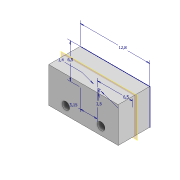
# Autodesk Inventor part: LimitSwitch
Saved by Autodesk Inventor 2022 (Build 260153000, 153)
## iProperties
Created: 2022-11-25
Part Number: LimitSwitch
Material: Generisch
Document SubType Name: Modeling
Designer: alexw
Density: 1 g/cm^3
Appearance: Vorgabe
Author: alexw
Autodesk Inventor part; units mm, degrees
ref_plane "YZ Plane" through (0, 0, 0) normal (1, 0, 0) x (0, 1, 0)
ref_plane "XZ Plane" through (0, 0, 0) normal (0, 1, 0) x (-1, 0, 0)
ref_plane "XY Plane" through (0, 0, 0) normal (0, 0, 1) x (1, 0, 0)
sketch "Skizze1" plane through (0, 0, 0) normal (0, 0, 1) x (1, 0, 0)
  line L0 (0, 0) -> (12.8, 0)
  line L1 (12.8, 0) -> (12.8, 6.5)
  line L2 (12.8, 6.5) -> (0, 6.5)
  line L3 (0, 6.5) -> (0, 0)
  circle A0 centre (3.15, 1.5) radius 0.7
  circle A1 centre (9.65, 1.5) radius 0.7
  line L4 (3.15, 1.5) -> (9.65, 1.5) construction
  line L5 (6.4, 0) -> (6.4, 6.5) construction
  dimension "d0" = 12.8
  dimension "d1" = 6.5
  dimension "d2" = 1.5
  dimension "d3" = 3.15
  dimension "d4" = 6.5
  dimension "d7" = 1.4
  constraints: 12 end point, 2 centre point, 2 horizontal, 2 midpoint, 2 parallel, 1 equal radius, 1 perpendicular
  measures "d0" distance of L1.end L2.end
  measures "d1" distance of L2.end L0.start
  measures "d2" distance from line of L4.start L0
  measures "d3" distance from line of L3 L4.start
  measures "d4" distance of L4.end L4.start
  measures "d7" diameter of A0
extrude "Extrusion1" add sketch "Skizze1" along normal blind 5.8
ref_plane "Arbeitsebene1" through (0, 0, 2.9) normal (0, 0, 1) x (1, 0, 0)
sketch "Skizze2" plane through (0, 0, 2.9) normal (0, 0, 1) x (1, 0, 0)
  circle A0 centre (3.15, 1.5) radius 0.7 construction
  line L0 (0, 0) -> (12.8, 0) projected
  line L1 (13.95, 8.3) -> (1, 6.5)
  line L2 (12.8, 6.5) -> (0, 6.5) projected
  line L3 (13.95, 11.5) -> (1, 6.5) construction
  line L4 (0, 6.5) -> (0, 0) projected
  line L5 (13.95, 8.3) -> (14.0188, 7.8048)
  line L6 (14.0188, 7.8048) -> (1.0688, 6.0048)
  line L7 (1.0688, 6.0048) -> (1, 6.5)
  point P0 (4.6318, 6.5)
  dimension "d8" = 10.8
  dimension "d9" = 10.8
  dimension "d10" = 8.3
  dimension "d11" = 11.5
  dimension "d12" = 1
  dimension "d13" = 0.5
  constraints: 10 end point, 3 perpendicular, 1 point on line
  measures "d8" horizontal distance of L3.start A0.centre
  measures "d9" horizontal distance of A0.centre L1.start
  measures "d10" distance from line of L1.start L0
  measures "d11" distance from line of L3.start L0
  measures "d12" distance from line of L4 L1.end
  measures "d13" distance between parallel lines of L6 L1
equation "\"d9\" = d8"
